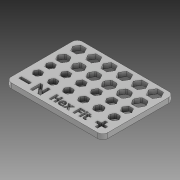
# Autodesk Inventor part: Standard Test Print
Saved by Autodesk Inventor 2022 (Build 260153000, 153)
## iProperties
Created: 2022-01-18
Part Number: Standard Test Print
Material: ABS Plastic
Document SubType Name: Modeling
Density: 1.06 g/cm^3
Appearance: Smooth - Medium Gray
Autodesk Inventor part; units mm, degrees
note: some values were not read from the file. Chosen so that the rebuilt part matches the saved one: direction of "Emboss1".
ref_plane "YZ Plane" through (0, 0, 0) normal (1, 0, 0) x (0, 1, 0)
ref_plane "XZ Plane" through (0, 0, 0) normal (0, 1, 0) x (-1, 0, 0)
ref_plane "XY Plane" through (0, 0, 0) normal (0, 0, 1) x (1, 0, 0)
sketch "Sketch1" plane through (0, 0, 0) normal (0, 1, 0) x (-1, 0, 0)
  line L0 (53.975, 34.925) -> (41.275, 34.925)
  line L1 (41.275, 34.925) -> (41.275, 31.75)
  line L2 (41.275, 31.75) -> (53.975, 31.75)
  line L3 (53.975, 31.75) -> (53.975, 34.925)
  line L4 (53.975, 34.925) -> (41.275, 31.75) construction
  line L5 (41.275, 34.925) -> (53.975, 31.75) construction
  line L6 (-41.275, 34.925) -> (-53.975, 34.925)
  line L7 (-53.975, 34.925) -> (-53.975, 31.75)
  line L8 (-53.975, 31.75) -> (-41.275, 31.75)
  line L9 (-41.275, 31.75) -> (-41.275, 34.925)
  line L10 (-41.275, 34.925) -> (-53.975, 31.75) construction
  line L11 (-53.975, 34.925) -> (-41.275, 31.75) construction
  line L12 (34.925, 39.6875) -> (34.925, 26.9875)
  line L13 (34.925, 26.9875) -> (31.75, 26.9875)
  line L14 (31.75, 26.9875) -> (25.4, 34.6945)
  line L15 (25.4, 34.6945) -> (25.4, 26.9875)
  line L16 (25.4, 26.9875) -> (22.225, 26.9875)
  line L17 (22.225, 26.9875) -> (22.225, 39.6875)
  line L18 (22.225, 39.6875) -> (25.4, 39.6875)
  line L19 (25.4, 39.6875) -> (31.75, 31.9805)
  line L20 (31.75, 31.9805) -> (31.75, 39.6875)
  line L21 (31.75, 39.6875) -> (34.925, 39.6875)
  line L22 (28.575, 35.834) -> (28.575, 30.841) construction
  line L23 (60.325, -44.45) -> (-60.325, -44.45)
  line L24 (-60.325, -44.45) -> (-60.325, 44.45)
  line L25 (-60.325, 44.45) -> (60.325, 44.45)
  line L26 (60.325, 44.45) -> (60.325, -44.45)
  line L27 (60.325, -44.45) -> (-60.325, 44.45) construction
  line L28 (-60.325, -44.45) -> (60.325, 44.45) construction
  line L29 (40.2927, -33.3375) -> (43.9588, -26.9875) construction
  line L30 (43.9588, -26.9875) -> (51.2912, -26.9875) construction
  line L31 (51.2912, -26.9875) -> (54.9573, -33.3375) construction
  line L32 (54.9573, -33.3375) -> (51.2912, -39.6875) construction
  line L33 (51.2912, -39.6875) -> (43.9588, -39.6875) construction
  line L34 (43.9588, -39.6875) -> (40.2927, -33.3375) construction
  line L35 (40.8082, -13.3945) -> (43.4432, -8.8305) construction
  line L36 (44.99, -7.9375) -> (50.26, -7.9375) construction
  line L37 (51.8068, -8.8305) -> (54.4418, -13.3945) construction
  line L38 (54.4418, -15.1805) -> (51.8068, -19.7445) construction
  line L39 (50.26, -20.6375) -> (44.99, -20.6375) construction
  line L40 (43.4432, -19.7445) -> (40.8082, -15.1805) construction
  arc A0 (43.4432, -19.7445) -> (44.99, -20.6375) centre (47.625, -14.2875) ccw construction
  arc A1 (40.8082, -13.3945) -> (40.8082, -15.1805) centre (47.625, -14.2875) ccw construction
  arc A2 (44.99, -7.9375) -> (43.4432, -8.8305) centre (47.625, -14.2875) ccw construction
  arc A3 (51.8068, -8.8305) -> (50.26, -7.9375) centre (47.625, -14.2875) ccw construction
  arc A4 (50.26, -20.6375) -> (51.8068, -19.7445) centre (47.625, -14.2875) ccw construction
  arc A5 (54.4418, -15.1805) -> (54.4418, -13.3945) centre (47.625, -14.2875) ccw construction
  line L41 (42.1257, 1.5875) -> (44.8754, 6.35) construction
  line L42 (44.8754, 6.35) -> (50.3746, 6.35) construction
  line L43 (50.3746, 6.35) -> (53.1243, 1.5875) construction
  line L44 (53.1243, 1.5875) -> (50.3746, -3.175) construction
  line L45 (50.3746, -3.175) -> (44.8754, -3.175) construction
  line L46 (44.8754, -3.175) -> (42.1257, 1.5875) construction
  line L47 (42.554, 18.2042) -> (44.4472, 21.4833) construction
  line L48 (45.7318, 22.225) -> (49.5182, 22.225) construction
  line L49 (50.8028, 21.4833) -> (52.696, 18.2042) construction
  line L50 (52.696, 16.7208) -> (50.8028, 13.4417) construction
  line L51 (49.5182, 12.7) -> (45.7318, 12.7) construction
  line L52 (44.4472, 13.4417) -> (42.554, 16.7208) construction
  arc A6 (44.4472, 13.4417) -> (45.7318, 12.7) centre (47.625, 17.4625) ccw construction
  arc A7 (42.554, 18.2042) -> (42.554, 16.7208) centre (47.625, 17.4625) ccw construction
  arc A8 (45.7318, 22.225) -> (44.4472, 21.4833) centre (47.625, 17.4625) ccw construction
  arc A9 (50.8028, 21.4833) -> (49.5182, 22.225) centre (47.625, 17.4625) ccw construction
  arc A10 (49.5182, 12.7) -> (50.8028, 13.4417) centre (47.625, 17.4625) ccw construction
  arc A11 (52.696, 16.7208) -> (52.696, 18.2042) centre (47.625, 17.4625) ccw construction
  arc A12 (30.4682, 12.7) -> (31.7528, 13.4417) centre (28.575, 17.4625) ccw
  line L53 (30.4682, 12.7) -> (26.6818, 12.7)
  arc A13 (25.3972, 13.4417) -> (26.6818, 12.7) centre (28.575, 17.4625) ccw
  line L54 (31.3246, 6.35) -> (34.0743, 1.5875)
  line L55 (25.8254, 6.35) -> (31.3246, 6.35)
  line L56 (34.0743, 1.5875) -> (31.3246, -3.175)
  line L57 (23.0757, 1.5875) -> (25.8254, 6.35)
  line L58 (31.3246, -3.175) -> (25.8254, -3.175)
  line L59 (25.8254, -3.175) -> (23.0757, 1.5875)
  line L60 (23.504, 18.2042) -> (25.3972, 21.4833)
  arc A14 (26.6818, 22.225) -> (25.3972, 21.4833) centre (28.575, 17.4625) ccw
  line L61 (21.2427, -33.3375) -> (24.9088, -26.9875)
  line L62 (32.2412, -26.9875) -> (35.9073, -33.3375)
  line L63 (35.9073, -33.3375) -> (32.2412, -39.6875)
  line L64 (32.2412, -39.6875) -> (24.9088, -39.6875)
  line L65 (24.9088, -39.6875) -> (21.2427, -33.3375)
  line L66 (24.9088, -26.9875) -> (32.2412, -26.9875)
  line L67 (31.21, -20.6375) -> (25.94, -20.6375)
  arc A15 (24.3932, -19.7445) -> (25.94, -20.6375) centre (28.575, -14.2875) ccw
  arc A16 (31.21, -20.6375) -> (32.7568, -19.7445) centre (28.575, -14.2875) ccw
  line L68 (24.3932, -19.7445) -> (21.7582, -15.1805)
  line L69 (35.3918, -15.1805) -> (32.7568, -19.7445)
  arc A17 (21.7582, -13.3945) -> (21.7582, -15.1805) centre (28.575, -14.2875) ccw
  arc A18 (35.3918, -15.1805) -> (35.3918, -13.3945) centre (28.575, -14.2875) ccw
  line L70 (21.7582, -13.3945) -> (24.3932, -8.8305)
  line L71 (32.7568, -8.8305) -> (35.3918, -13.3945)
  arc A19 (25.94, -7.9375) -> (24.3932, -8.8305) centre (28.575, -14.2875) ccw
  line L72 (25.94, -7.9375) -> (31.21, -7.9375)
  arc A20 (32.7568, -8.8305) -> (31.21, -7.9375) centre (28.575, -14.2875) ccw
  arc A21 (23.504, 18.2042) -> (23.504, 16.7208) centre (28.575, 17.4625) ccw
  line L73 (25.3972, 13.4417) -> (23.504, 16.7208)
  line L74 (33.646, 16.7208) -> (31.7528, 13.4417)
  arc A22 (33.646, 16.7208) -> (33.646, 18.2042) centre (28.575, 17.4625) ccw
  line L75 (31.7528, 21.4833) -> (33.646, 18.2042)
  line L76 (26.6818, 22.225) -> (30.4682, 22.225)
  arc A23 (31.7528, 21.4833) -> (30.4682, 22.225) centre (28.575, 17.4625) ccw
  arc A24 (11.4182, 12.7) -> (12.7028, 13.4417) centre (9.525, 17.4625) ccw construction
  line L77 (11.4182, 12.7) -> (7.6318, 12.7) construction
  arc A25 (6.3472, 13.4417) -> (7.6318, 12.7) centre (9.525, 17.4625) ccw construction
  line L78 (12.2746, 6.35) -> (15.0243, 1.5875) construction
  line L79 (6.7754, 6.35) -> (12.2746, 6.35) construction
  line L80 (15.0243, 1.5875) -> (12.2746, -3.175) construction
  line L81 (4.0257, 1.5875) -> (6.7754, 6.35) construction
  line L82 (12.2746, -3.175) -> (6.7754, -3.175) construction
  line L83 (6.7754, -3.175) -> (4.0257, 1.5875) construction
  line L84 (4.454, 18.2042) -> (6.3472, 21.4833) construction
  arc A26 (7.6318, 22.225) -> (6.3472, 21.4833) centre (9.525, 17.4625) ccw construction
  line L85 (2.1927, -33.3375) -> (5.8588, -26.9875) construction
  line L86 (13.1912, -26.9875) -> (16.8573, -33.3375) construction
  line L87 (16.8573, -33.3375) -> (13.1912, -39.6875) construction
  line L88 (13.1912, -39.6875) -> (5.8588, -39.6875) construction
  line L89 (5.8588, -39.6875) -> (2.1927, -33.3375) construction
  line L90 (5.8588, -26.9875) -> (13.1912, -26.9875) construction
  line L91 (12.16, -20.6375) -> (6.89, -20.6375) construction
  arc A27 (5.3432, -19.7445) -> (6.89, -20.6375) centre (9.525, -14.2875) ccw construction
  arc A28 (12.16, -20.6375) -> (13.7068, -19.7445) centre (9.525, -14.2875) ccw construction
  line L92 (5.3432, -19.7445) -> (2.7082, -15.1805) construction
  line L93 (16.3418, -15.1805) -> (13.7068, -19.7445) construction
  arc A29 (2.7082, -13.3945) -> (2.7082, -15.1805) centre (9.525, -14.2875) ccw construction
  arc A30 (16.3418, -15.1805) -> (16.3418, -13.3945) centre (9.525, -14.2875) ccw construction
  line L94 (2.7082, -13.3945) -> (5.3432, -8.8305) construction
  line L95 (13.7068, -8.8305) -> (16.3418, -13.3945) construction
  arc A31 (6.89, -7.9375) -> (5.3432, -8.8305) centre (9.525, -14.2875) ccw construction
  line L96 (6.89, -7.9375) -> (12.16, -7.9375) construction
  arc A32 (13.7068, -8.8305) -> (12.16, -7.9375) centre (9.525, -14.2875) ccw construction
  arc A33 (4.454, 18.2042) -> (4.454, 16.7208) centre (9.525, 17.4625) ccw construction
  line L97 (6.3472, 13.4417) -> (4.454, 16.7208) construction
  line L98 (14.596, 16.7208) -> (12.7028, 13.4417) construction
  arc A34 (14.596, 16.7208) -> (14.596, 18.2042) centre (9.525, 17.4625) ccw construction
  line L99 (12.7028, 21.4833) -> (14.596, 18.2042) construction
  line L100 (7.6318, 22.225) -> (11.4182, 22.225) construction
  arc A35 (12.7028, 21.4833) -> (11.4182, 22.225) centre (9.525, 17.4625) ccw construction
  arc A36 (-7.6318, 12.7) -> (-6.3472, 13.4417) centre (-9.525, 17.4625) ccw construction
  line L101 (-7.6318, 12.7) -> (-11.4182, 12.7) construction
  arc A37 (-12.7028, 13.4417) -> (-11.4182, 12.7) centre (-9.525, 17.4625) ccw construction
  line L102 (-6.7754, 6.35) -> (-4.0257, 1.5875) construction
  line L103 (-12.2746, 6.35) -> (-6.7754, 6.35) construction
  line L104 (-4.0257, 1.5875) -> (-6.7754, -3.175) construction
  line L105 (-15.0243, 1.5875) -> (-12.2746, 6.35) construction
  line L106 (-6.7754, -3.175) -> (-12.2746, -3.175) construction
  line L107 (-12.2746, -3.175) -> (-15.0243, 1.5875) construction
  line L108 (-14.596, 18.2042) -> (-12.7028, 21.4833) construction
  arc A38 (-11.4182, 22.225) -> (-12.7028, 21.4833) centre (-9.525, 17.4625) ccw construction
  line L109 (-16.8573, -33.3375) -> (-13.1912, -26.9875) construction
  line L110 (-5.8588, -26.9875) -> (-2.1927, -33.3375) construction
  line L111 (-2.1927, -33.3375) -> (-5.8588, -39.6875) construction
  line L112 (-5.8588, -39.6875) -> (-13.1912, -39.6875) construction
  line L113 (-13.1912, -39.6875) -> (-16.8573, -33.3375) construction
  line L114 (-13.1912, -26.9875) -> (-5.8588, -26.9875) construction
  line L115 (-6.89, -20.6375) -> (-12.16, -20.6375) construction
  arc A39 (-13.7068, -19.7445) -> (-12.16, -20.6375) centre (-9.525, -14.2875) ccw construction
  arc A40 (-6.89, -20.6375) -> (-5.3432, -19.7445) centre (-9.525, -14.2875) ccw construction
  line L116 (-13.7068, -19.7445) -> (-16.3418, -15.1805) construction
  line L117 (-2.7082, -15.1805) -> (-5.3432, -19.7445) construction
  arc A41 (-16.3418, -13.3945) -> (-16.3418, -15.1805) centre (-9.525, -14.2875) ccw construction
  arc A42 (-2.7082, -15.1805) -> (-2.7082, -13.3945) centre (-9.525, -14.2875) ccw construction
  line L118 (-16.3418, -13.3945) -> (-13.7068, -8.8305) construction
  line L119 (-5.3432, -8.8305) -> (-2.7082, -13.3945) construction
  arc A43 (-12.16, -7.9375) -> (-13.7068, -8.8305) centre (-9.525, -14.2875) ccw construction
  line L120 (-12.16, -7.9375) -> (-6.89, -7.9375) construction
  arc A44 (-5.3432, -8.8305) -> (-6.89, -7.9375) centre (-9.525, -14.2875) ccw construction
  arc A45 (-14.596, 18.2042) -> (-14.596, 16.7208) centre (-9.525, 17.4625) ccw construction
  line L121 (-12.7028, 13.4417) -> (-14.596, 16.7208) construction
  line L122 (-4.454, 16.7208) -> (-6.3472, 13.4417) construction
  arc A46 (-4.454, 16.7208) -> (-4.454, 18.2042) centre (-9.525, 17.4625) ccw construction
  line L123 (-6.3472, 21.4833) -> (-4.454, 18.2042) construction
  line L124 (-11.4182, 22.225) -> (-7.6318, 22.225) construction
  arc A47 (-6.3472, 21.4833) -> (-7.6318, 22.225) centre (-9.525, 17.4625) ccw construction
  arc A48 (-26.6818, 12.7) -> (-25.3972, 13.4417) centre (-28.575, 17.4625) ccw construction
  line L125 (-26.6818, 12.7) -> (-30.4682, 12.7) construction
  arc A49 (-31.7528, 13.4417) -> (-30.4682, 12.7) centre (-28.575, 17.4625) ccw construction
  line L126 (-25.8254, 6.35) -> (-23.0757, 1.5875) construction
  line L127 (-31.3246, 6.35) -> (-25.8254, 6.35) construction
  line L128 (-23.0757, 1.5875) -> (-25.8254, -3.175) construction
  line L129 (-34.0743, 1.5875) -> (-31.3246, 6.35) construction
  line L130 (-25.8254, -3.175) -> (-31.3246, -3.175) construction
  line L131 (-31.3246, -3.175) -> (-34.0743, 1.5875) construction
  line L132 (-33.646, 18.2042) -> (-31.7528, 21.4833) construction
  arc A50 (-30.4682, 22.225) -> (-31.7528, 21.4833) centre (-28.575, 17.4625) ccw construction
  line L133 (-35.9073, -33.3375) -> (-32.2412, -26.9875) construction
  line L134 (-24.9088, -26.9875) -> (-21.2427, -33.3375) construction
  line L135 (-21.2427, -33.3375) -> (-24.9088, -39.6875) construction
  line L136 (-24.9088, -39.6875) -> (-32.2412, -39.6875) construction
  line L137 (-32.2412, -39.6875) -> (-35.9073, -33.3375) construction
  line L138 (-32.2412, -26.9875) -> (-24.9088, -26.9875) construction
  line L139 (-25.94, -20.6375) -> (-31.21, -20.6375) construction
  arc A51 (-32.7568, -19.7445) -> (-31.21, -20.6375) centre (-28.575, -14.2875) ccw construction
  arc A52 (-25.94, -20.6375) -> (-24.3932, -19.7445) centre (-28.575, -14.2875) ccw construction
  line L140 (-32.7568, -19.7445) -> (-35.3918, -15.1805) construction
  line L141 (-21.7582, -15.1805) -> (-24.3932, -19.7445) construction
  arc A53 (-35.3918, -13.3945) -> (-35.3918, -15.1805) centre (-28.575, -14.2875) ccw construction
  arc A54 (-21.7582, -15.1805) -> (-21.7582, -13.3945) centre (-28.575, -14.2875) ccw construction
  line L142 (-35.3918, -13.3945) -> (-32.7568, -8.8305) construction
  line L143 (-24.3932, -8.8305) -> (-21.7582, -13.3945) construction
  arc A55 (-31.21, -7.9375) -> (-32.7568, -8.8305) centre (-28.575, -14.2875) ccw construction
  line L144 (-31.21, -7.9375) -> (-25.94, -7.9375) construction
  arc A56 (-24.3932, -8.8305) -> (-25.94, -7.9375) centre (-28.575, -14.2875) ccw construction
  arc A57 (-33.646, 18.2042) -> (-33.646, 16.7208) centre (-28.575, 17.4625) ccw construction
  line L145 (-31.7528, 13.4417) -> (-33.646, 16.7208) construction
  line L146 (-23.504, 16.7208) -> (-25.3972, 13.4417) construction
  arc A58 (-23.504, 16.7208) -> (-23.504, 18.2042) centre (-28.575, 17.4625) ccw construction
  line L147 (-25.3972, 21.4833) -> (-23.504, 18.2042) construction
  line L148 (-30.4682, 22.225) -> (-26.6818, 22.225) construction
  arc A59 (-25.3972, 21.4833) -> (-26.6818, 22.225) centre (-28.575, 17.4625) ccw construction
  arc A60 (-45.7318, 12.7) -> (-44.4472, 13.4417) centre (-47.625, 17.4625) ccw construction
  line L149 (-45.7318, 12.7) -> (-49.5182, 12.7) construction
  arc A61 (-50.8028, 13.4417) -> (-49.5182, 12.7) centre (-47.625, 17.4625) ccw construction
  line L150 (-44.8754, 6.35) -> (-42.1257, 1.5875) construction
  line L151 (-50.3746, 6.35) -> (-44.8754, 6.35) construction
  line L152 (-42.1257, 1.5875) -> (-44.8754, -3.175) construction
  line L153 (-53.1243, 1.5875) -> (-50.3746, 6.35) construction
  line L154 (-44.8754, -3.175) -> (-50.3746, -3.175) construction
  line L155 (-50.3746, -3.175) -> (-53.1243, 1.5875) construction
  line L156 (-52.696, 18.2042) -> (-50.8028, 21.4833) construction
  arc A62 (-49.5182, 22.225) -> (-50.8028, 21.4833) centre (-47.625, 17.4625) ccw construction
  line L157 (-54.9573, -33.3375) -> (-51.2912, -26.9875) construction
  line L158 (-43.9588, -26.9875) -> (-40.2927, -33.3375) construction
  line L159 (-40.2927, -33.3375) -> (-43.9588, -39.6875) construction
  line L160 (-43.9588, -39.6875) -> (-51.2912, -39.6875) construction
  line L161 (-51.2912, -39.6875) -> (-54.9573, -33.3375) construction
  line L162 (-51.2912, -26.9875) -> (-43.9588, -26.9875) construction
  line L163 (-44.99, -20.6375) -> (-50.26, -20.6375) construction
  arc A63 (-51.8068, -19.7445) -> (-50.26, -20.6375) centre (-47.625, -14.2875) ccw construction
  arc A64 (-44.99, -20.6375) -> (-43.4432, -19.7445) centre (-47.625, -14.2875) ccw construction
  line L164 (-51.8068, -19.7445) -> (-54.4418, -15.1805) construction
  line L165 (-40.8082, -15.1805) -> (-43.4432, -19.7445) construction
  arc A65 (-54.4418, -13.3945) -> (-54.4418, -15.1805) centre (-47.625, -14.2875) ccw construction
  arc A66 (-40.8082, -15.1805) -> (-40.8082, -13.3945) centre (-47.625, -14.2875) ccw construction
  line L166 (-54.4418, -13.3945) -> (-51.8068, -8.8305) construction
  line L167 (-43.4432, -8.8305) -> (-40.8082, -13.3945) construction
  arc A67 (-50.26, -7.9375) -> (-51.8068, -8.8305) centre (-47.625, -14.2875) ccw construction
  line L168 (-50.26, -7.9375) -> (-44.99, -7.9375) construction
  arc A68 (-43.4432, -8.8305) -> (-44.99, -7.9375) centre (-47.625, -14.2875) ccw construction
  arc A69 (-52.696, 18.2042) -> (-52.696, 16.7208) centre (-47.625, 17.4625) ccw construction
  line L169 (-50.8028, 13.4417) -> (-52.696, 16.7208) construction
  line L170 (-42.554, 16.7208) -> (-44.4472, 13.4417) construction
  arc A70 (-42.554, 16.7208) -> (-42.554, 18.2042) centre (-47.625, 17.4625) ccw construction
  line L171 (-44.4472, 21.4833) -> (-42.554, 18.2042) construction
  line L172 (-49.5182, 22.225) -> (-45.7318, 22.225) construction
  arc A71 (-44.4472, 21.4833) -> (-45.7318, 22.225) centre (-47.625, 17.4625) ccw construction
  line L173 (44.0321, -39.5605) -> (51.2179, -39.5605)
  line L174 (51.2179, -39.5605) -> (54.8107, -33.3375)
  line L175 (54.8107, -33.3375) -> (51.2179, -27.1145)
  line L176 (51.2179, -27.1145) -> (44.0321, -27.1145)
  line L177 (44.0321, -27.1145) -> (40.4393, -33.3375)
  line L178 (40.4393, -33.3375) -> (44.0321, -39.5605)
  line L179 (45.0154, -20.5105) -> (50.2346, -20.5105)
  arc A72 (50.2346, -20.5105) -> (51.7095, -19.6589) centre (47.625, -14.2875) ccw
  line L180 (51.7095, -19.6589) -> (54.3191, -15.1391)
  arc A73 (54.3191, -15.1391) -> (54.3191, -13.4359) centre (47.625, -14.2875) ccw
  line L181 (54.3191, -13.4359) -> (51.7095, -8.9161)
  arc A74 (51.7095, -8.9161) -> (50.2346, -8.0645) centre (47.625, -14.2875) ccw
  line L182 (50.2346, -8.0645) -> (45.0154, -8.0645)
  arc A75 (45.0154, -8.0645) -> (43.5405, -8.9161) centre (47.625, -14.2875) ccw
  line L183 (43.5405, -8.9161) -> (40.9309, -13.4359)
  arc A76 (40.9309, -13.4359) -> (40.9309, -15.1391) centre (47.625, -14.2875) ccw
  line L184 (40.9309, -15.1391) -> (43.5405, -19.6589)
  arc A77 (43.5405, -19.6589) -> (45.0154, -20.5105) centre (47.625, -14.2875) ccw
  line L185 (44.9487, -3.048) -> (50.3013, -3.048)
  line L186 (50.3013, -3.048) -> (52.9776, 1.5875)
  line L187 (52.9776, 1.5875) -> (50.3013, 6.223)
  line L188 (50.3013, 6.223) -> (44.9487, 6.223)
  line L189 (44.9487, 6.223) -> (42.2724, 1.5875)
  line L190 (42.2724, 1.5875) -> (44.9487, -3.048)
  line L191 (42.6762, 16.7631) -> (44.5449, 13.5264)
  arc A78 (44.5449, 13.5264) -> (45.7563, 12.827) centre (47.625, 17.4625) ccw
  line L192 (45.7563, 12.827) -> (49.4937, 12.827)
  arc A79 (49.4937, 12.827) -> (50.7051, 13.5264) centre (47.625, 17.4625) ccw
  line L193 (50.7051, 13.5264) -> (52.5738, 16.7631)
  arc A80 (52.5738, 16.7631) -> (52.5738, 18.1619) centre (47.625, 17.4625) ccw
  line L194 (52.5738, 18.1619) -> (50.7051, 21.3986)
  arc A81 (50.7051, 21.3986) -> (49.4937, 22.098) centre (47.625, 17.4625) ccw
  line L195 (49.4937, 22.098) -> (45.7563, 22.098)
  arc A82 (45.7563, 22.098) -> (44.5449, 21.3986) centre (47.625, 17.4625) ccw
  line L196 (44.5449, 21.3986) -> (42.6762, 18.1619)
  arc A83 (42.6762, 18.1619) -> (42.6762, 16.7631) centre (47.625, 17.4625) ccw
  line L197 (13.2645, -39.8145) -> (17.004, -33.3375)
  line L198 (17.004, -33.3375) -> (13.2645, -26.8605)
  line L199 (13.2645, -26.8605) -> (5.7855, -26.8605)
  line L200 (5.7855, -26.8605) -> (2.046, -33.3375)
  line L201 (2.046, -33.3375) -> (5.7855, -39.8145)
  line L202 (5.7855, -39.8145) -> (13.2645, -39.8145)
  line L203 (13.8042, -19.8298) -> (16.4643, -15.2222)
  arc A84 (16.4643, -15.2222) -> (16.4643, -13.3528) centre (9.525, -14.2875) ccw
  line L204 (16.4643, -13.3528) -> (13.8042, -8.7452)
  arc A85 (13.8042, -8.7452) -> (12.1852, -7.8105) centre (9.525, -14.2875) ccw
  line L205 (12.1852, -7.8105) -> (6.8648, -7.8105)
  arc A86 (6.8648, -7.8105) -> (5.2458, -8.7452) centre (9.525, -14.2875) ccw
  line L206 (5.2458, -8.7452) -> (2.5857, -13.3528)
  arc A87 (2.5857, -13.3528) -> (2.5857, -15.2222) centre (9.525, -14.2875) ccw
  line L207 (2.5857, -15.2222) -> (5.2458, -19.8298)
  arc A88 (5.2458, -19.8298) -> (6.8648, -20.7645) centre (9.525, -14.2875) ccw
  line L208 (6.8648, -20.7645) -> (12.1852, -20.7645)
  arc A89 (12.1852, -20.7645) -> (13.8042, -19.8298) centre (9.525, -14.2875) ccw
  line L209 (-5.7122, -39.9415) -> (-1.8994, -33.3375)
  line L210 (-1.8994, -33.3375) -> (-5.7122, -26.7335)
  line L211 (-5.7122, -26.7335) -> (-13.3378, -26.7335)
  line L212 (-13.3378, -26.7335) -> (-17.1506, -33.3375)
  line L213 (-17.1506, -33.3375) -> (-13.3378, -39.9415)
  line L214 (-13.3378, -39.9415) -> (-5.7122, -39.9415)
  line L215 (-5.1483, -19.9149) -> (-2.4632, -15.2641)
  arc A90 (-2.4632, -15.2641) -> (-2.4632, -13.3109) centre (-9.525, -14.2875) ccw
  line L216 (-2.4632, -13.3109) -> (-5.1483, -8.6601)
  arc A91 (-5.1483, -8.6601) -> (-6.8399, -7.6835) centre (-9.525, -14.2875) ccw
  line L217 (-6.8399, -7.6835) -> (-12.2101, -7.6835)
  arc A92 (-12.2101, -7.6835) -> (-13.9017, -8.6601) centre (-9.525, -14.2875) ccw
  line L218 (-13.9017, -8.6601) -> (-16.5868, -13.3109)
  arc A93 (-16.5868, -13.3109) -> (-16.5868, -15.2641) centre (-9.525, -14.2875) ccw
  line L219 (-16.5868, -15.2641) -> (-13.9017, -19.9149)
  arc A94 (-13.9017, -19.9149) -> (-12.2101, -20.8915) centre (-9.525, -14.2875) ccw
  line L220 (-12.2101, -20.8915) -> (-6.8399, -20.8915)
  arc A95 (-6.8399, -20.8915) -> (-5.1483, -19.9149) centre (-9.525, -14.2875) ccw
  line L221 (-24.1007, -19.9998) -> (-21.3909, -15.3062)
  arc A96 (-21.3909, -15.3062) -> (-21.3909, -13.2688) centre (-28.575, -14.2875) ccw
  line L222 (-21.3909, -13.2688) -> (-24.1007, -8.5752)
  arc A97 (-24.1007, -8.5752) -> (-25.8652, -7.5565) centre (-28.575, -14.2875) ccw
  line L223 (-25.8652, -7.5565) -> (-31.2848, -7.5565)
  arc A98 (-31.2848, -7.5565) -> (-33.0493, -8.5752) centre (-28.575, -14.2875) ccw
  line L224 (-33.0493, -8.5752) -> (-35.7591, -13.2688)
  arc A99 (-35.7591, -13.2688) -> (-35.7591, -15.3062) centre (-28.575, -14.2875) ccw
  line L225 (-35.7591, -15.3062) -> (-33.0493, -19.9998)
  arc A100 (-33.0493, -19.9998) -> (-31.2848, -21.0185) centre (-28.575, -14.2875) ccw
  line L226 (-31.2848, -21.0185) -> (-25.8652, -21.0185)
  arc A101 (-25.8652, -21.0185) -> (-24.1007, -19.9998) centre (-28.575, -14.2875) ccw
  line L227 (-32.4611, -26.6065) -> (-36.3473, -33.3375)
  line L228 (-36.3473, -33.3375) -> (-32.4611, -40.0685)
  line L229 (-32.4611, -40.0685) -> (-24.6889, -40.0685)
  line L230 (-24.6889, -40.0685) -> (-20.8027, -33.3375)
  line L231 (-20.8027, -33.3375) -> (-24.6889, -26.6065)
  line L232 (-24.6889, -26.6065) -> (-32.4611, -26.6065)
  line L233 (-51.5845, -26.4795) -> (-55.5439, -33.3375)
  line L234 (-55.5439, -33.3375) -> (-51.5845, -40.1955)
  line L235 (-51.5845, -40.1955) -> (-43.6655, -40.1955)
  line L236 (-43.6655, -40.1955) -> (-39.7061, -33.3375)
  line L237 (-39.7061, -33.3375) -> (-43.6655, -26.4795)
  line L238 (-43.6655, -26.4795) -> (-51.5845, -26.4795)
  line L239 (-54.9314, -15.3485) -> (-52.197, -20.0845)
  arc A102 (-52.197, -20.0845) -> (-50.3593, -21.1455) centre (-47.625, -14.2875) ccw
  line L240 (-50.3593, -21.1455) -> (-44.8907, -21.1455)
  arc A103 (-44.8907, -21.1455) -> (-43.053, -20.0845) centre (-47.625, -14.2875) ccw
  line L241 (-43.053, -20.0845) -> (-40.3186, -15.3485)
  arc A104 (-40.3186, -15.3485) -> (-40.3186, -13.2265) centre (-47.625, -14.2875) ccw
  line L242 (-40.3186, -13.2265) -> (-43.053, -8.4905)
  arc A105 (-43.053, -8.4905) -> (-44.8907, -7.4295) centre (-47.625, -14.2875) ccw
  line L243 (-44.8907, -7.4295) -> (-50.3593, -7.4295)
  arc A106 (-50.3593, -7.4295) -> (-52.197, -8.4905) centre (-47.625, -14.2875) ccw
  line L244 (-52.197, -8.4905) -> (-54.9314, -13.2265)
  arc A107 (-54.9314, -13.2265) -> (-54.9314, -15.3485) centre (-47.625, -14.2875) ccw
  line L245 (12.348, 6.477) -> (6.702, 6.477)
  line L246 (6.702, 6.477) -> (3.8791, 1.5875)
  line L247 (3.8791, 1.5875) -> (6.702, -3.302)
  line L248 (6.702, -3.302) -> (12.348, -3.302)
  line L249 (12.348, -3.302) -> (15.1709, 1.5875)
  line L250 (15.1709, 1.5875) -> (12.348, 6.477)
  line L251 (4.3319, 16.6782) -> (6.2493, 13.3573)
  arc A108 (6.2493, 13.3573) -> (7.6076, 12.573) centre (9.525, 17.4625) ccw
  line L252 (7.6076, 12.573) -> (11.4424, 12.573)
  arc A109 (11.4424, 12.573) -> (12.8007, 13.3573) centre (9.525, 17.4625) ccw
  line L253 (12.8007, 13.3573) -> (14.7181, 16.6782)
  arc A110 (14.7181, 16.6782) -> (14.7181, 18.2468) centre (9.525, 17.4625) ccw
  line L254 (14.7181, 18.2468) -> (12.8007, 21.5677)
  arc A111 (12.8007, 21.5677) -> (11.4424, 22.352) centre (9.525, 17.4625) ccw
  line L255 (11.4424, 22.352) -> (7.6076, 22.352)
  arc A112 (7.6076, 22.352) -> (6.2493, 21.5677) centre (9.525, 17.4625) ccw
  line L256 (6.2493, 21.5677) -> (4.3319, 18.2468)
  arc A113 (4.3319, 18.2468) -> (4.3319, 16.6782) centre (9.525, 17.4625) ccw
  line L257 (-6.6287, 6.604) -> (-12.4213, 6.604)
  line L258 (-12.4213, 6.604) -> (-15.3176, 1.5875)
  line L259 (-15.3176, 1.5875) -> (-12.4213, -3.429)
  line L260 (-12.4213, -3.429) -> (-6.6287, -3.429)
  line L261 (-6.6287, -3.429) -> (-3.7324, 1.5875)
  line L262 (-3.7324, 1.5875) -> (-6.6287, 6.604)
  line L263 (-6.1512, 13.2731) -> (-4.21, 16.6354)
  arc A114 (-4.21, 16.6354) -> (-4.21, 18.2896) centre (-9.525, 17.4625) ccw
  line L264 (-4.21, 18.2896) -> (-6.1512, 21.6519)
  arc A115 (-6.1512, 21.6519) -> (-7.5838, 22.479) centre (-9.525, 17.4625) ccw
  line L265 (-7.5838, 22.479) -> (-11.4662, 22.479)
  arc A116 (-11.4662, 22.479) -> (-12.8988, 21.6519) centre (-9.525, 17.4625) ccw
  line L266 (-12.8988, 21.6519) -> (-14.84, 18.2896)
  arc A117 (-14.84, 18.2896) -> (-14.84, 16.6354) centre (-9.525, 17.4625) ccw
  line L267 (-14.84, 16.6354) -> (-12.8988, 13.2731)
  arc A118 (-12.8988, 13.2731) -> (-11.4662, 12.446) centre (-9.525, 17.4625) ccw
  line L268 (-11.4662, 12.446) -> (-7.5838, 12.446)
  arc A119 (-7.5838, 12.446) -> (-6.1512, 13.2731) centre (-9.525, 17.4625) ccw
  line L269 (-31.5446, 6.731) -> (-34.5142, 1.5875)
  line L270 (-34.5142, 1.5875) -> (-31.5446, -3.556)
  line L271 (-31.5446, -3.556) -> (-25.6054, -3.556)
  line L272 (-25.6054, -3.556) -> (-22.6358, 1.5875)
  line L273 (-22.6358, 1.5875) -> (-25.6054, 6.731)
  line L274 (-25.6054, 6.731) -> (-31.5446, 6.731)
  line L275 (-44.5821, 6.858) -> (-50.6679, 6.858)
  line L276 (-50.6679, 6.858) -> (-53.7108, 1.5875)
  line L277 (-53.7108, 1.5875) -> (-50.6679, -3.683)
  line L278 (-50.6679, -3.683) -> (-44.5821, -3.683)
  line L279 (-44.5821, -3.683) -> (-41.5392, 1.5875)
  line L280 (-41.5392, 1.5875) -> (-44.5821, 6.858)
  line L281 (-49.6131, 12.192) -> (-45.6369, 12.192)
  arc A120 (-45.6369, 12.192) -> (-44.0547, 13.1055) centre (-47.625, 17.4625) ccw
  line L282 (-44.0547, 13.1055) -> (-42.0666, 16.549)
  arc A121 (-42.0666, 16.549) -> (-42.0666, 18.376) centre (-47.625, 17.4625) ccw
  line L283 (-42.0666, 18.376) -> (-44.0547, 21.8195)
  arc A122 (-44.0547, 21.8195) -> (-45.6369, 22.733) centre (-47.625, 17.4625) ccw
  line L284 (-45.6369, 22.733) -> (-49.6131, 22.733)
  arc A123 (-49.6131, 22.733) -> (-51.1953, 21.8195) centre (-47.625, 17.4625) ccw
  line L285 (-51.1953, 21.8195) -> (-53.1834, 18.376)
  arc A124 (-53.1834, 18.376) -> (-53.1834, 16.549) centre (-47.625, 17.4625) ccw
  line L286 (-53.1834, 16.549) -> (-51.1953, 13.1055)
  arc A125 (-51.1953, 13.1055) -> (-49.6131, 12.192) centre (-47.625, 17.4625) ccw
  line L287 (-30.5398, 12.319) -> (-26.6102, 12.319)
  arc A126 (-26.6102, 12.319) -> (-25.103, 13.1892) centre (-28.575, 17.4625) ccw
  line L288 (-25.103, 13.1892) -> (-23.1382, 16.5923)
  arc A127 (-23.1382, 16.5923) -> (-23.1382, 18.3327) centre (-28.575, 17.4625) ccw
  line L289 (-23.1382, 18.3327) -> (-25.103, 21.7358)
  arc A128 (-25.103, 21.7358) -> (-26.6102, 22.606) centre (-28.575, 17.4625) ccw
  line L290 (-26.6102, 22.606) -> (-30.5398, 22.606)
  arc A129 (-30.5398, 22.606) -> (-32.047, 21.7358) centre (-28.575, 17.4625) ccw
  line L291 (-32.047, 21.7358) -> (-34.0118, 18.3327)
  arc A130 (-34.0118, 18.3327) -> (-34.0118, 16.5923) centre (-28.575, 17.4625) ccw
  line L292 (-34.0118, 16.5923) -> (-32.047, 13.1892)
  arc A131 (-32.047, 13.1892) -> (-30.5398, 12.319) centre (-28.575, 17.4625) ccw
  line L293 (-49.2125, 26.9875) -> (-46.0375, 26.9875)
  line L294 (-46.0375, 26.9875) -> (-46.0375, 39.6875)
  line L295 (-46.0375, 39.6875) -> (-49.2125, 39.6875)
  line L296 (-49.2125, 39.6875) -> (-49.2125, 26.9875)
  line L297 (-49.2125, 26.9875) -> (-46.0375, 39.6875) construction
  line L298 (-46.0375, 26.9875) -> (-49.2125, 39.6875) construction
  line L299 (16.7692, 31.5145) -> (-35.8192, 31.5145) construction
  line L300 (-35.8192, 31.5145) -> (-35.8192, 35.1605) construction
  line L301 (-35.8192, 35.1605) -> (16.7692, 35.1605) construction
  line L302 (16.7692, 35.1605) -> (16.7692, 31.5145) construction
  line L303 (4.7278, 38.2196) -> (7.1206, 38.2196)
  line L304 (7.1206, 38.2196) -> (7.1206, 33.9975)
  line L305 (7.1206, 33.9975) -> (10.3702, 33.9975)
  line L306 (10.3702, 33.9975) -> (10.3702, 38.2196)
  line L307 (10.3702, 38.2196) -> (12.763, 38.2196)
  line L308 (12.763, 38.2196) -> (12.763, 28.6946)
  line L309 (12.763, 28.6946) -> (10.3702, 28.6946)
  line L310 (10.3702, 28.6946) -> (10.3702, 32.1835)
  line L311 (10.3702, 32.1835) -> (7.1206, 32.1835)
  line L312 (7.1206, 32.1835) -> (7.1206, 28.6946)
  line L313 (7.1206, 28.6946) -> (4.7278, 28.6946)
  line L314 (4.7278, 28.6946) -> (4.7278, 38.2196)
  spline S0 degree 2 poles (-0.7989, 38.4126) (1.2389, 38.4126) (3.4079, 36.4675) (3.4079, 34.669) knots 0 0 0 1 2 2 2
  spline S1 degree 2 poles (3.4079, 34.669) (3.4079, 32.9091) (1.3855, 30.8096) (-0.4361, 30.8096) knots 0 0 0 1 2 2 2
  spline S2 degree 2 poles (-0.4361, 30.8096) (-2.0802, 30.8096) (-3.7475, 32.5926) (-3.7475, 34.2445) knots 0 0 0 1 2 2 2
  line L315 (-3.7475, 34.2445) -> (-3.7475, 35.0549)
  line L316 (-3.7475, 35.0549) -> (1.1694, 35.0549)
  spline S3 degree 2 poles (1.1694, 35.0549) (1.1385, 35.5567) (0.7757, 36.2205) (0.4824, 36.4212) knots 0 0 0 1 2 2 2
  spline S4 degree 2 poles (0.4824, 36.4212) (0.1968, 36.6218) (-0.5751, 36.7917) (-1.0305, 36.7917) knots 0 0 0 1 2 2 2
  spline S5 degree 2 poles (-1.0305, 36.7917) (-1.4164, 36.7917) (-2.1728, 36.6218) (-2.4893, 36.4752) knots 0 0 0 1 2 2 2
  spline S6 degree 2 poles (-2.4893, 36.4752) (-2.7672, 36.3594) (-3.2303, 36.0738) (-3.377, 35.9658) knots 0 0 0 1 2 2 2
  line L317 (-3.377, 35.9658) -> (-3.6163, 35.9658)
  line L318 (-3.6163, 35.9658) -> (-3.6163, 37.8183)
  spline S7 degree 2 poles (-3.6163, 37.8183) (-3.3384, 37.9263) (-2.8907, 38.1116) (-2.4893, 38.2042) knots 0 0 0 1 2 2 2
  spline S8 degree 2 poles (-2.4893, 38.2042) (-2.1265, 38.3045) (-1.3546, 38.4126) (-0.7989, 38.4126) knots 0 0 0 1 2 2 2
  spline S9 degree 2 poles (-1.5399, 33.7041) (-1.5245, 32.994) (-0.8992, 32.2453) (-0.2586, 32.2453) knots 0 0 0 1 2 2 2
  spline S10 degree 2 poles (-0.2586, 32.2453) (0.3975, 32.2453) (1.1385, 33.0326) (1.1771, 33.7041) knots 0 0 0 1 2 2 2
  line L319 (1.1771, 33.7041) -> (-1.5399, 33.7041)
  line L320 (-11.9834, 38.2196) -> (-9.359, 38.2196)
  line L321 (-9.359, 38.2196) -> (-7.9928, 36.1587)
  line L322 (-7.9928, 36.1587) -> (-6.588, 38.2196)
  line L323 (-6.588, 38.2196) -> (-4.0176, 38.2196)
  line L324 (-4.0176, 38.2196) -> (-6.6652, 34.6227)
  line L325 (-6.6652, 34.6227) -> (-4.0639, 31.0334)
  line L326 (-4.0639, 31.0334) -> (-6.6883, 31.0334)
  line L327 (-6.6883, 31.0334) -> (-8.0314, 33.0558)
  line L328 (-8.0314, 33.0558) -> (-9.3822, 31.0334)
  line L329 (-9.3822, 31.0334) -> (-11.9526, 31.0334)
  line L330 (-11.9526, 31.0334) -> (-9.3513, 34.5686)
  line L331 (-9.3513, 34.5686) -> (-11.9834, 38.2196)
  line L332 (-23.1603, 30.5086) -> (-19.1619, 30.5086)
  line L333 (-19.1619, 30.5086) -> (-19.1619, 32.307)
  line L334 (-19.1619, 32.307) -> (-22.8438, 32.307)
  line L335 (-22.8438, 32.307) -> (-22.8438, 34.121)
  line L336 (-22.8438, 34.121) -> (-19.1619, 34.121)
  line L337 (-19.1619, 34.121) -> (-19.1619, 38.2196)
  line L338 (-19.1619, 38.2196) -> (-16.7845, 38.2196)
  line L339 (-16.7845, 38.2196) -> (-16.7845, 28.6946)
  line L340 (-16.7845, 28.6946) -> (-23.1603, 28.6946)
  line L341 (-23.1603, 28.6946) -> (-23.1603, 30.5086)
  line L342 (-26.5025, 38.2196) -> (-24.264, 38.2196)
  line L343 (-24.264, 38.2196) -> (-24.264, 31.0334)
  line L344 (-24.264, 31.0334) -> (-26.5025, 31.0334)
  line L345 (-26.5025, 31.0334) -> (-26.5025, 38.2196)
  line L346 (-26.572, 30.0068) -> (-24.2023, 30.0068)
  line L347 (-24.2023, 30.0068) -> (-24.2023, 28.2624)
  line L348 (-24.2023, 28.2624) -> (-26.572, 28.2624)
  line L349 (-26.572, 28.2624) -> (-26.572, 30.0068)
  spline S11 degree 2 poles (-30.964, 38.3586) (-29.5977, 38.3586) (-28.3473, 37.2316) (-28.3473, 35.9503) knots 0 0 0 1 2 2 2
  line L350 (-28.3473, 35.9503) -> (-28.3473, 32.5926)
  line L351 (-28.3473, 32.5926) -> (-27.4905, 32.5926)
  line L352 (-27.4905, 32.5926) -> (-27.4905, 31.0334)
  line L353 (-27.4905, 31.0334) -> (-28.3473, 31.0334)
  line L354 (-28.3473, 31.0334) -> (-28.3473, 28.9802)
  line L355 (-28.3473, 28.9802) -> (-30.5857, 28.9802)
  line L356 (-30.5857, 28.9802) -> (-30.5857, 31.0334)
  line L357 (-30.5857, 31.0334) -> (-32.747, 31.0334)
  line L358 (-32.747, 31.0334) -> (-32.747, 32.5926)
  line L359 (-32.747, 32.5926) -> (-30.5857, 32.5926)
  line L360 (-30.5857, 32.5926) -> (-30.5857, 35.1476)
  spline S12 degree 2 poles (-30.5857, 35.1476) (-30.5857, 35.5258) (-30.6012, 36.0893) (-30.6938, 36.3131) knots 0 0 0 1 2 2 2
  spline S13 degree 2 poles (-30.6938, 36.3131) (-30.7864, 36.5369) (-31.2418, 36.7994) (-31.6741, 36.7994) knots 0 0 0 1 2 2 2
  spline S14 degree 2 poles (-31.6741, 36.7994) (-31.8593, 36.7994) (-32.4383, 36.645) (-32.554, 36.5833) knots 0 0 0 1 2 2 2
  line L361 (-32.554, 36.5833) -> (-32.747, 36.5833)
  line L362 (-32.747, 36.5833) -> (-32.747, 38.1579)
  spline S15 degree 2 poles (-32.747, 38.1579) (-32.3842, 38.2505) (-31.566, 38.3586) (-30.964, 38.3586) knots 0 0 0 1 2 2 2
  point P0 (47.625, 33.3375)
  point P1 (-47.625, 33.3375)
  point P2 (-47.625, 33.3375)
  point P3 (47.625, 33.3375)
  point P4 (-47.625, 33.3375)
  point P5 (47.625, 33.3375)
  point P6 (28.575, 33.3375)
  point P7 (0, 0)
  point P8 (47.625, -33.3375)
  point P9 (47.625, 1.5875)
  point P10 (28.575, 1.5875)
  point P11 (28.575, -33.3375)
  point P12 (9.525, 1.5875)
  point P13 (9.525, -33.3375)
  point P14 (-9.525, 1.5875)
  point P15 (-9.525, -33.3375)
  point P16 (-28.575, 1.5875)
  point P17 (-28.575, -33.3375)
  point P18 (-47.625, 1.5875)
  point P19 (-47.625, -33.3375)
  point P20 (-49.2125, 34.925)
  point P21 (-46.0375, 34.925)
  point P22 (-46.0375, 31.75)
  point P23 (-49.2125, 31.75)
  point P24 (-9.525, 31.5145)
  point P25 (-35.8192, 33.3375)
  point P26 (-47.625, 33.3375)
  dimension "d33" = 12.7
  dimension "d34" = 3.175
  dimension "d61" = 12.7
  dimension "d62" = 12.7
  dimension "d64" = 3.175
  dimension "d79" = 12.7
  dimension "d80" = 12.7
  dimension "d82" = 13.75
  dimension "d83" = 19.05
  dimension "d84" = 9.525
  dimension "d85" = 9.525
  dimension "d86" = 10.25
  dimension "d87" = 15.875
  dimension "d88" = 15.875
  dimension "d93" = 19.05
  dimension "d98" = 0.127
  dimension "d99" = 0.127
  dimension "d100" = 0.127
  dimension "d101" = 0.127
  dimension "d102" = 0.127
  dimension "d103" = 0.127
  dimension "d104" = 0.127
  dimension "d105" = 0.127
  dimension "d106" = 0.254
  dimension "d107" = 0.254
  dimension "d108" = 0.254
  dimension "d109" = 0.254
  dimension "d110" = 0.381
  dimension "d111" = 0.381
  dimension "d112" = 0.381
  dimension "d113" = 0.381
  dimension "d114" = 0.508
  dimension "d115" = 0.508
  dimension "d116" = 0.508
  dimension "d117" = 0.508
  dimension "d118" = 15.875
  dimension "d119" = 66.675
  dimension "d120" = 33.3375
  dimension "d121" = 88.9
  dimension "d122" = 19.05
  dimension "d123" = 9.525
  dimension "d124" = 120.65
  constraints: 599 end point, 264 point on circle, 132 centre point, 18 midpoint, 12 coincident, 11 parallel, 10 concentric, 10 horizontal, 7 equal length, 7 perpendicular, 7 vertical alignment, 6 point on line, 3 horizontal alignment, 1 vertical, 592 other
  measures "d33" distance of L1.end L2.end
  measures "d34" distance of L2.end L0.start
  measures "d61" distance between parallel lines of L17 L12
  measures "d62" distance between parallel lines of L18 L16
  measures "d64" distance between parallel lines of L19 L14
  measures "d79" distance between parallel lines of L30 L33
  measures "d80" distance between parallel lines of L36 L39
  measures "d82" diameter of A5
  measures "d83" distance of point (47.625, -14.287) point (47.625, -33.337)
  measures "d84" distance between parallel lines of L42 L45
  measures "d85" distance between parallel lines of L48 L51
  measures "d86" diameter of A11
  measures "d87" distance of point (47.625, 17.463) point (47.625, 1.588)
  measures "d88" distance of point (47.625, 1.588) point (47.625, -14.287)
  measures "d93" distance of L51.start L53.start
  measures "d98" distance between parallel lines of L33 L173
  measures "d99" distance between parallel lines of L179 L39
  measures "d100" distance between parallel lines of L45 L185
  measures "d101" distance between parallel lines of L51 L192
  measures "d102" distance between parallel lines of L88 L202
  measures "d103" distance between parallel lines of L91 L208
  measures "d104" distance between parallel lines of L82 L248
  measures "d105" distance between parallel lines of L77 L252
  measures "d106" distance between parallel lines of L112 L214
  measures "d107" distance between parallel lines of L220 L115
  measures "d108" distance between parallel lines of L260 L106
  measures "d109" distance between parallel lines of L268 L101
  measures "d110" distance between parallel lines of L229 L136
  measures "d111" distance between parallel lines of L226 L139
  measures "d112" distance between parallel lines of L271 L130
  measures "d113" distance between parallel lines of L287 L125
  measures "d114" distance between parallel lines of L235 L160
  measures "d115" distance between parallel lines of L240 L163
  measures "d116" distance between parallel lines of L278 L154
  measures "d117" distance between parallel lines of L281 L149
  measures "d118" distance of A7.centre point (47.625, 33.338)
  measures "d119" distance of point (47.625, 33.338) point (47.625, -33.337)
  measures "d120" vertical distance of point (47.625, -33.337) point (0, 0)
  measures "d121" distance of L25.end L23.start
  measures "d122" distance of point (-9.525, -33.337) point (9.525, -33.337)
  measures "d123" horizontal distance of point (9.525, -33.337) point (0, 0)
  measures "d124" distance of L23.start L23.end
extrude "Extrusion1" add sketch "Sketch1" against normal blind 6.35 contours L23 L24 L25 L26 | L303 L304 L305 L306 L307 L308 L309 L310 L311 L312 L313 L314 | S0 S1 S2 L315 L316 S3 S4 S5 S6 L317 L318 S7 S8 | L319 S10 S9 | L320 L321 L322 L323 L324 L325 L326 L327 L328 L329 L330 L331 | L332 L333 L334 L335 L336 L337 L338 L339 L340 L341 | L342 L343 L344 L345 | L346 L347 L348 L349 | S11 L350 L351 L352 L353 L354 L355 L356 L357 L358 L359 L360 S12 S13 S14 L361 L362 S15
fillet "Fillet1" radius 6.35 4 edges at (-60.325, -3.175, 44.45) (-60.325, -3.175, -44.45) (60.325, -3.175, -44.45) (60.325, -3.175, 44.45)
fillet "Fillet2" radius 0.3969 26 edges at (-25.4, -3.175, 34.6945) (53.975, -3.175, 31.75) (53.975, -3.175, 34.925) (41.275, -3.175, 34.925) (41.275, -3.175, 31.75) (-25.4, -3.175, 26.9875) (-22.225, -3.175, 26.9875) (-22.225, -3.175, 39.6875) (-25.4, -3.175, 39.6875) (-31.75, -3.175, 31.9805) (-31.75, -3.175, 26.9875) (-34.925, -3.175, 26.9875) (-31.75, -3.175, 39.6875) (-34.925, -3.175, 39.6875) (-41.275, -3.175, 34.925) (-41.275, -3.175, 31.75) (-53.975, -3.175, 31.75) (-53.975, -3.175, 34.925) (46.0375, -3.175, 31.75) (49.2125, -3.175, 31.75) (49.2125, -3.175, 26.9875) (46.0375, -3.175, 26.9875) (46.0375, -3.175, 39.6875) (46.0375, -3.175, 34.925) (49.2125, -3.175, 39.6875) (49.2125, -3.175, 34.925)
chamfer "Chamfer1" distance 0.7937 angle 45 216 edges at (-53.0143, -6.35, -36.449) (-53.0143, -6.35, -30.226) (-47.625, -6.35, -39.5605) (-42.2357, -6.35, -36.449) (-42.2357, -6.35, -30.226) (-47.625, -6.35, -27.1145) (-34.0743, -6.35, -36.5125) (-28.575, -6.35, -39.6875) (-23.0757, -6.35, -36.5125) (-23.0757, -6.35, -30.1625) (-28.575, -6.35, -26.9875) (-34.0743, -6.35, -30.1625) (-15.1342, -6.35, -36.576) (-9.525, -6.35, -39.8145) (-3.9158, -6.35, -36.576) (-3.9158, -6.35, -30.099) (-9.525, -6.35, -26.8605) (-15.1342, -6.35, -30.099) (3.8058, -6.35, -36.6395) (9.525, -6.35, -39.9415) (15.2442, -6.35, -36.6395) (15.2442, -6.35, -30.0355) (9.525, -6.35, -26.7335) (3.8058, -6.35, -30.0355) (22.7458, -6.35, -36.703) (28.575, -6.35, -40.0685) (34.4042, -6.35, -36.703) (34.4042, -6.35, -29.972) (22.7458, -6.35, -29.972) (28.575, -6.35, -26.6065) (41.6858, -6.35, -36.7665) (47.625, -6.35, -40.1955) (53.5642, -6.35, -36.7665) (53.5642, -6.35, -29.9085) (47.625, -6.35, -26.4795) (41.6858, -6.35, -29.9085) (41.6858, -6.35, -17.7165) (43.9335, -6.35, -20.6814) (47.625, -6.35, -21.1455) (51.3165, -6.35, -20.6814) (53.5642, -6.35, -17.7165) (55.008, -6.35, -14.2875) (51.3165, -6.35, -7.8936) (47.625, -6.35, -7.4295) (43.9335, -6.35, -7.8936) (40.242, -6.35, -14.2875) (41.6858, -6.35, -10.8585) (34.4042, -6.35, -10.922) (32.203, -6.35, -8.0036) (28.575, -6.35, -7.5565) (22.7458, -6.35, -10.922) (24.947, -6.35, -8.0036) (21.319, -6.35, -14.2875) (22.7458, -6.35, -17.653) (24.947, -6.35, -20.5714) (28.575, -6.35, -21.0185) (32.203, -6.35, -20.5714) (34.4042, -6.35, -17.653) (35.831, -6.35, -14.2875) (15.2442, -6.35, -17.5895) (13.0895, -6.35, -20.4614) (9.525, -6.35, -20.8915) (5.9605, -6.35, -20.4614) (3.8058, -6.35, -17.5895) (2.396, -6.35, -14.2875) (9.525, -6.35, -7.6835) (5.9605, -6.35, -8.1136) (3.8058, -6.35, -10.9855) (13.0895, -6.35, -8.1136) (15.2442, -6.35, -10.9855) (16.654, -6.35, -14.2875) (50.4415, -6.35, 22.3408) (47.625, -6.35, 22.733) (44.8085, -6.35, 22.3408) (43.0606, -6.35, 20.0978) (41.992, -6.35, 17.4625) (43.0606, -6.35, 14.8273) (44.8085, -6.35, 12.5842) (47.625, -6.35, 12.192) (50.4415, -6.35, 12.5842) (52.1894, -6.35, 14.8272) (53.258, -6.35, 17.4625) (52.1894, -6.35, 20.0978) (43.0606, -6.35, 4.2228) (43.0606, -6.35, -1.0477) (47.625, -6.35, -3.683) (52.1894, -6.35, -1.0477) (52.1894, -6.35, 4.2228) (47.625, -6.35, 6.858) (33.0294, -6.35, 4.1593) (33.0294, -6.35, -0.9842) (28.575, -6.35, -3.556) (24.1206, -6.35, -0.9842) (24.1206, -6.35, 4.1593) (28.575, -6.35, 6.731) (28.575, -6.35, 12.319) (25.822, -6.35, 12.6942) (24.1206, -6.35, 14.8908) (23.069, -6.35, 17.4625) (24.1206, -6.35, 20.0343) (31.328, -6.35, 22.2308) (28.575, -6.35, 22.606) (33.0294, -6.35, 20.0343) (34.081, -6.35, 17.4625) (33.0294, -6.35, 14.8907) (31.328, -6.35, 12.6942) (13.8694, -6.35, 4.0958) (13.8694, -6.35, -0.9207) (9.525, -6.35, -3.429) (5.1806, -6.35, -0.9207) (5.1806, -6.35, 4.0958) (9.525, -6.35, 6.604) (6.8355, -6.35, 12.8041) (5.1806, -6.35, 14.9543) (4.146, -6.35, 17.4625) (5.1806, -6.35, 19.9708) (6.8355, -6.35, 22.1209) (9.525, -6.35, 22.479) (12.2145, -6.35, 22.1209) (13.8694, -6.35, 19.9708) (14.904, -6.35, 17.4625) (13.8694, -6.35, 14.9543) (12.2145, -6.35, 12.8041) (9.525, -6.35, 12.446) (25.822, -6.35, 22.2308) (-5.2906, -6.35, 4.0323) (-9.525, -6.35, 6.477) (-13.7594, -6.35, 4.0323) (-13.7594, -6.35, -0.8572) (-9.525, -6.35, -3.302) (-5.2906, -6.35, -0.8572) (-13.7594, -6.35, 15.0177) (-12.151, -6.35, 12.9141) (-9.525, -6.35, 12.573) (-6.899, -6.35, 12.9141) (-5.2906, -6.35, 15.0177) (-4.273, -6.35, 17.4625) (-5.2906, -6.35, 19.9073) (-6.899, -6.35, 22.0109) (-9.525, -6.35, 22.352) (-12.151, -6.35, 22.0109) (-13.7594, -6.35, 19.9073) (-14.777, -6.35, 17.4625) (-9.525, -6.35, -7.8105) (-13.026, -6.35, -8.2236) (-15.1342, -6.35, -11.049) (-16.527, -6.35, -14.2875) (-15.1342, -6.35, -17.526) (-13.026, -6.35, -20.3514) (-9.525, -6.35, -20.7645) (-6.024, -6.35, -20.3514) (-3.9158, -6.35, -17.526) (-2.523, -6.35, -14.2875) (-3.9158, -6.35, -11.049) (-6.024, -6.35, -8.2236) (-32.6994, -6.35, -0.7938) (-28.575, -6.35, -3.175) (-24.4506, -6.35, -0.7937) (-24.4506, -6.35, 3.9687) (-28.575, -6.35, 6.35) (-32.6994, -6.35, 3.9687) (-43.6105, -6.35, 3.9053) (-47.625, -6.35, 6.223) (-51.6395, -6.35, 3.9053) (-51.6395, -6.35, -0.7302) (-47.625, -6.35, -3.048) (-43.6105, -6.35, -0.7302) (-35.45, -6.35, -14.2875) (-34.0743, -6.35, -17.4625) (-32.0125, -6.35, -20.2414) (-25.1375, -6.35, -20.2414) (-28.575, -6.35, -20.6375) (-34.0743, -6.35, -11.1125) (-32.0125, -6.35, -8.3336) (-28.575, -6.35, -7.9375) (-25.1375, -6.35, -8.3336) (-23.0757, -6.35, -11.1125) (-21.7, -6.35, -14.2875) (-23.0757, -6.35, -17.4625) (-53.0143, -6.35, -17.399) (-47.625, -6.35, -8.0645) (-53.0143, -6.35, -11.176) (-54.373, -6.35, -14.2875) (-50.999, -6.35, -8.4436) (-44.251, -6.35, -8.4436) (-42.2357, -6.35, -11.176) (-40.877, -6.35, -14.2875) (-42.2357, -6.35, -17.399) (-44.251, -6.35, -20.1314) (-47.625, -6.35, -20.5105) (-50.999, -6.35, -20.1314) (-28.575, -6.35, 12.7) (-26.0125, -6.35, 13.0241) (-24.4506, -6.35, 15.0813) (-23.45, -6.35, 17.4625) (-24.4506, -6.35, 19.8438) (-26.0125, -6.35, 21.9009) (-32.6994, -6.35, 19.8438) (-31.1375, -6.35, 21.9009) (-28.575, -6.35, 22.225) (-33.7, -6.35, 17.4625) (-32.6994, -6.35, 15.0813) (-31.1375, -6.35, 13.0241) (-51.6395, -6.35, 15.1448) (-50.124, -6.35, 13.1341) (-47.625, -6.35, 12.827) (-45.126, -6.35, 13.1341) (-43.6105, -6.35, 15.1448) (-42.627, -6.35, 17.4625) (-43.6105, -6.35, 19.7803) (-45.126, -6.35, 21.7909) (-47.625, -6.35, 22.098) (-50.124, -6.35, 21.7909) (-51.6395, -6.35, 19.7803) (-52.623, -6.35, 17.4625) (53.5642, -6.35, -10.8585)
chamfer "Chamfer2" distance 0.3969 angle 45 52 edges at (43.6563, -6.35, 34.925) (41.3912, -6.35, 34.8088) (41.275, -6.35, 33.3375) (41.3912, -6.35, 31.8662) (43.6563, -6.35, 31.75) (45.9213, -6.35, 31.6338) (46.0375, -6.35, 29.3687) (46.1537, -6.35, 27.1037) (47.625, -6.35, 26.9875) (49.0963, -6.35, 27.1037) (49.2125, -6.35, 29.3687) (49.3287, -6.35, 31.6338) (51.5938, -6.35, 31.75) (53.8588, -6.35, 31.8662) (53.975, -6.35, 33.3375) (53.8588, -6.35, 34.8088) (51.5938, -6.35, 34.925) (49.3287, -6.35, 35.0412) (49.2125, -6.35, 37.3063) (49.0963, -6.35, 39.5713) (47.625, -6.35, 39.6875) (46.1537, -6.35, 39.5713) (46.0375, -6.35, 37.3063) (45.9213, -6.35, 35.0412) (-22.225, -6.35, 33.3375) (-22.3412, -6.35, 39.5713) (-23.9173, -6.35, 39.6875) (-25.3821, -6.35, 39.6496) (-28.2829, -6.35, 36.1885) (-31.4872, -6.35, 32.7128) (-31.75, -6.35, 36.1885) (-31.8662, -6.35, 39.5713) (-33.3375, -6.35, 39.6875) (-34.8088, -6.35, 39.5713) (-34.925, -6.35, 33.3375) (-34.8088, -6.35, 27.1037) (-33.2327, -6.35, 26.9875) (-31.7679, -6.35, 27.0254) (-28.8671, -6.35, 30.4865) (-25.6628, -6.35, 33.9622) (-25.4, -6.35, 30.4865) (-25.2838, -6.35, 27.1037) (-23.8125, -6.35, 26.9875) (-22.3412, -6.35, 27.1037) (-47.625, -6.35, 31.75) (-41.3912, -6.35, 31.8662) (-41.275, -6.35, 33.3375) (-41.3912, -6.35, 34.8088) (-47.625, -6.35, 34.925) (-53.8588, -6.35, 34.8088) (-53.975, -6.35, 33.3375) (-53.8588, -6.35, 31.8662)
emboss "Emboss1" sketch "Sketch1" operation cut depth 3.175 direction (0, -1, 0) contours L303 L304 L305 L306 L307 L308 L309 L310 L311 L312 L313 L314 | S0 S1 S2 L315 L316 S3 S4 S5 S6 L317 L318 S7 S8 | L320 L321 L322 L323 L324 L325 L326 L327 L328 L329 L330 L331 | L332 L333 L334 L335 L336 L337 L338 L339 L340 L341 | L342 L343 L344 L345 | L346 L347 L348 L349 | S11 L350 L351 L352 L353 L354 L355 L356 L357 L358 L359 L360 S12 S13 S14 L361 L362 S15
body "Solid1"
